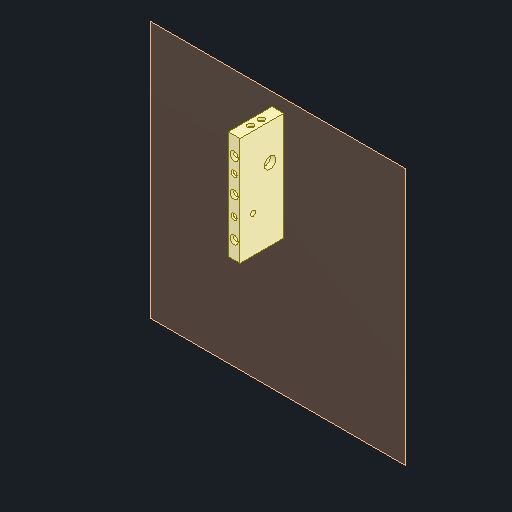
# Autodesk Inventor part: middle_gear_holder
Saved by Autodesk Inventor 2023 (Build 270158000, 158)
## iProperties
Created: 2024-04-23
Part Number: middle_gear_holder
Material: Nylon 6/6
Document SubType Name: Modeling
Designer: szymo
Density: 1.13 g/cm^3
Appearance: Nylon 6
Mass: 25.6721 g
Surface Area: 95.1123 cm^2
Volume: 22.7187 cm^3
Author: szymo
Autodesk Inventor part; units mm, degrees
ref_plane "YZ Plane" through (0, 0, 0) normal (1, 0, 0) x (0, 1, 0)
ref_plane "XZ Plane" through (0, 0, 0) normal (0, 1, 0) x (-1, 0, 0)
ref_plane "XY Plane" through (0, 0, 0) normal (0, 0, 1) x (1, 0, 0)
ref_plane "Work Plane1" through (0, 0, 0) normal (0, 0, 1) x (1, 0, 0)
ref_plane "Work Plane2" through (-89, -40.3889, 33.5) normal (0, 0, 1) x (1, 0, 0)
sketch "Sketch1" plane through (0, 0, 0) normal (0, 0, 1) x (1, 0, 0)
  line L0 (23.5, 88.5) -> (-23.5, 88.5) projected
  line L1 (-23.5, 88.5) -> (-23.5, 36.5) projected
  line L2 (-26.5, 33.5) -> (-89, 33.5) projected
  line L3 (-89, 33.5) -> (-89, -72.5) projected
  line L4 (-89, -72.5) -> (-77, -72.5) projected
  line L5 (-74, -75.5) -> (-74, -93.5) projected
  line L6 (-74, -93.5) -> (74, -93.5) projected
  line L7 (74, -93.5) -> (74, -75.5) projected
  line L8 (77, -72.5) -> (89, -72.5) projected
  line L9 (89, -72.5) -> (89, 33.5) projected
  line L10 (89, 33.5) -> (26.5, 33.5) projected
  line L11 (23.5, 36.5) -> (23.5, 88.5) projected
  line L12 (-4.5, 81.5) -> (-4.5, 36.5) projected
  line L13 (-7.5, 33.5) -> (-13.5, 33.5) projected
  line L14 (-16.5, 36.5) -> (-16.5, 81.5) projected
  line L15 (7.5, 84.5) -> (13.5, 84.5) projected
  line L16 (16.5, 81.5) -> (16.5, 36.5) projected
  line L17 (13.5, 33.5) -> (7.5, 33.5) projected
  line L18 (4.5, 36.5) -> (4.5, 81.5) projected
  line L19 (-13.5, 84.5) -> (-7.5, 84.5) projected
  line L20 (-4.5, 88.5) -> (4.5, 88.5)
  line L21 (4.5, 88.5) -> (4.5, 5.75)
  line L22 (4.5, 5.75) -> (-4.5, 5.75)
  line L23 (-4.5, 5.75) -> (-4.5, 88.5)
  line L24 (-32.2, 4.75) -> (-59.9, 4.75)
  arc A0 (13.5, 33.5) -> (16.5, 36.5) centre (13.5, 36.5) ccw projected
  arc A1 (4.5, 36.5) -> (7.5, 33.5) centre (7.5, 36.5) ccw projected
  arc A2 (7.5, 84.5) -> (4.5, 81.5) centre (7.5, 81.5) ccw projected
  arc A3 (16.5, 81.5) -> (13.5, 84.5) centre (13.5, 81.5) ccw projected
  arc A4 (-4.5, 81.5) -> (-7.5, 84.5) centre (-7.5, 81.5) ccw projected
  arc A5 (-7.5, 33.5) -> (-4.5, 36.5) centre (-7.5, 36.5) ccw projected
  arc A6 (-16.5, 36.5) -> (-13.5, 33.5) centre (-13.5, 36.5) ccw projected
  arc A7 (-13.5, 84.5) -> (-16.5, 81.5) centre (-13.5, 81.5) ccw projected
  arc A8 (-26.5, 33.5) -> (-23.5, 36.5) centre (-26.5, 36.5) ccw projected
  arc A9 (-74, -75.5) -> (-77, -72.5) centre (-77, -75.5) ccw projected
  arc A10 (77, -72.5) -> (74, -75.5) centre (77, -75.5) ccw projected
  arc A11 (23.5, 36.5) -> (26.5, 33.5) centre (26.5, 36.5) ccw projected
  circle A12 centre (39.125, 25.9125) radius 1.0065 projected
  circle A13 centre (72.95, 12.275) radius 1.0065 projected
  circle A14 centre (86, 30.5) radius 1.0065 projected
  circle A15 centre (-86, 30.5) radius 1.0065 projected
  circle A16 centre (-39.125, 12.3375) radius 1.0065 projected
  circle A17 centre (-72.95, 25.975) radius 1.0065 projected
  circle A18 centre (-72.95, 12.275) radius 1.0065 projected
  circle A19 centre (-39.125, 25.9125) radius 1.0065 projected
  circle A20 centre (-86, 7.75) radius 1.0065 projected
  circle A21 centre (86, 7.75) radius 1.0065 projected
  circle A22 centre (72.95, 25.975) radius 1.0065 projected
  circle A23 centre (39.125, 12.3375) radius 1.0065 projected
  circle A24 centre (-24.1, -73.1) radius 1.2295 projected
  circle A25 centre (-42.4984, -44.6666) radius 1.2295 projected
  circle A26 centre (-79, -42.3889) radius 1.2295 projected
  circle A27 centre (-19.5, 28.875) radius 1.2295 projected
  circle A28 centre (19.5, 9.55) radius 1.2295 projected
  circle A29 centre (19.5, 47.3) radius 1.2295 projected
  circle A30 centre (-19.5, 47.3) radius 1.2295 projected
  circle A31 centre (0, 74.7) radius 1.2295 projected
  circle A32 centre (-19.4231, 74.8077) radius 1.2295 projected
  circle A33 centre (19.5, 74.7) radius 1.2295 projected
  circle A34 centre (0, 49.05) radius 1.2295 projected
  circle A35 centre (19.5, 28.875) radius 1.2295 projected
  circle A36 centre (0, 19.125) radius 1.2295 projected
  circle A37 centre (-19.5, 9.55) radius 1.2295 projected
  circle A38 centre (24.1, -73.1) radius 1.2295 projected
  circle A39 centre (42.5, -44.6649) radius 1.2295 projected
  circle A40 centre (79, -42.3889) radius 1.2295 projected
  circle A41 centre (21.5, -85.5) radius 1.8 projected
  circle A42 centre (-64.5, -85.5) radius 1.8 projected
  circle A43 centre (-83.4, -19.2889) radius 1.8 projected
  circle A44 centre (-21.5, -85.5) radius 1.8 projected
  circle A45 centre (64.5, -85.5) radius 1.8 projected
  line L25 (-58.2315, -77.6013) -> (-77.7685, -63.3434) projected
  line L26 (-79, -36.3889) -> (-79, 1.75) projected
  line L27 (-75.7766, -45.4056) -> (-47.1423, -47.5438) projected
  line L28 (-21.1, -26.5751) -> (-21.1, -22.0255) projected
  line L29 (-46.9357, -41.5592) -> (-76, -39.3889) projected
  line L30 (-79, -60.9201) -> (-79, -48.3972) projected
  line L31 (32.0924, 4.75) -> (76, 4.75) projected
  line L32 (79, 1.75) -> (79, -36.3889) projected
  line L33 (76, -39.3889) -> (46.9371, -41.5577) projected
  line L34 (21.1, -22.0255) -> (21.1, -26.5749) projected
  line L35 (47.144, -47.5423) -> (76, -45.3889) projected
  line L36 (79, -48.3889) -> (79, -60.9201) projected
  line L37 (77.7685, -63.3434) -> (58.2315, -77.6013) projected
  line L38 (57, -80.0246) -> (57, -87.5) projected
  arc A46 (55, -89.5) -> (57, -87.5) centre (55, -87.5) ccw projected
  line L39 (55, -89.5) -> (31, -89.5) projected
  arc A47 (29, -87.5) -> (31, -89.5) centre (31, -87.5) ccw projected
  line L40 (29, -87.5) -> (29, -79.2522) projected
  line L41 (14, -79.5039) -> (14, -87.5) projected
  arc A48 (12, -89.5) -> (14, -87.5) centre (12, -87.5) ccw projected
  line L42 (12, -89.5) -> (-12, -89.5) projected
  arc A49 (-14, -87.5) -> (-12, -89.5) centre (-12, -87.5) ccw projected
  line L43 (-14, -87.5) -> (-14, -79.5039) projected
  line L44 (-29, -79.2522) -> (-29, -87.5) projected
  arc A50 (-31, -89.5) -> (-29, -87.5) centre (-31, -87.5) ccw projected
  line L45 (-31, -89.5) -> (-55, -89.5) projected
  arc A51 (-57, -87.5) -> (-55, -89.5) centre (-55, -87.5) ccw projected
  line L46 (-57, -87.5) -> (-57, -80.0246) projected
  line L47 (-66.95, 28.9125) -> (-45.125, 28.9125) projected
  line L48 (-42.125, 25.9125) -> (-42.125, 12.275) projected
  line L49 (-45.125, 9.275) -> (-66.95, 9.275) projected
  line L50 (-69.95, 12.275) -> (-69.95, 25.9125) projected
  line L51 (-16.5, 12.75) -> (-16.5, 25.5) projected
  line L52 (-13.5, 28.5) -> (-7.5, 28.5) projected
  line L53 (-4.5, 25.5) -> (-4.5, 12.75) projected
  line L54 (-7.5, 9.75) -> (-13.5, 9.75) projected
  line L55 (66.95, 9.3375) -> (45.125, 9.3375) projected
  line L56 (42.125, 12.3375) -> (42.125, 25.975) projected
  line L57 (45.125, 28.975) -> (66.95, 28.975) projected
  line L58 (69.95, 25.975) -> (69.95, 12.3375) projected
  line L59 (4.5, 12.75) -> (4.5, 25.5) projected
  line L60 (7.5, 28.5) -> (13.5, 28.5) projected
  line L61 (16.5, 25.5) -> (16.5, 12.75) projected
  line L62 (13.5, 9.75) -> (7.5, 9.75) projected
  line L63 (44.5181, -40.6102) -> (28.0046, -22.8717) projected
  line L64 (27.2109, -20.577) -> (29.1029, 2.0005) projected
  line L65 (-44.7206, -49.1201) -> (-29.3549, -77.8368) projected
  line L66 (-76, 4.75) -> (-32.0924, 4.75) projected
  line L67 (-29.1029, 2.0005) -> (-27.2109, -20.5772) projected
  line L68 (-28.0044, -22.8717) -> (-44.5164, -40.6115) projected
  line L69 (29.3549, -77.8368) -> (44.7222, -49.1185) projected
  line L70 (-14.6042, -77.6983) -> (-37.8537, -46.8489) projected
  line L71 (-37.4786, -42.8259) -> (-22.0793, -28.7924) projected
  line L72 (-21.1105, -21.775) -> (-23.0609, 1.4995) projected
  line L73 (-20.0714, 4.75) -> (20.0714, 4.75) projected
  line L74 (23.0609, 1.4995) -> (21.1105, -21.775) projected
  line L75 (22.0795, -28.7925) -> (37.4798, -42.8243) projected
  line L76 (37.8551, -46.8475) -> (14.6042, -77.6983) projected
  circle A52 centre (-78, -67.1725) radius 1.2295 projected
  arc A53 (76, -39.3889) -> (79, -36.3889) centre (76, -36.3889) ccw projected
  arc A54 (44.5181, -40.6102) -> (46.9371, -41.5577) centre (46.7138, -38.566) ccw projected
  arc A55 (27.2109, -20.577) -> (28.0046, -22.8717) centre (30.2004, -20.8276) ccw projected
  arc A56 (32.0924, 4.75) -> (29.1029, 2.0005) centre (32.0924, 1.75) ccw projected
  arc A57 (79, 1.75) -> (76, 4.75) centre (76, 1.75) ccw projected
  arc A58 (-42.125, 25.9125) -> (-45.125, 28.9125) centre (-45.125, 25.9125) ccw projected
  arc A59 (-45.125, 9.275) -> (-42.125, 12.275) centre (-45.125, 12.275) ccw projected
  arc A60 (-69.95, 12.275) -> (-66.95, 9.275) centre (-66.95, 12.275) ccw projected
  arc A61 (-66.95, 28.9125) -> (-69.95, 25.9125) centre (-66.95, 25.9125) ccw projected
  arc A62 (-13.5, 28.5) -> (-16.5, 25.5) centre (-13.5, 25.5) ccw projected
  arc A63 (-4.5, 25.5) -> (-7.5, 28.5) centre (-7.5, 25.5) ccw projected
  arc A64 (-7.5, 9.75) -> (-4.5, 12.75) centre (-7.5, 12.75) ccw projected
  arc A65 (-16.5, 12.75) -> (-13.5, 9.75) centre (-13.5, 12.75) ccw projected
  arc A66 (58.2315, -77.6013) -> (57, -80.0246) centre (60, -80.0246) ccw projected
  arc A67 (29.3549, -77.8368) -> (29, -79.2522) centre (32, -79.2522) ccw projected
  arc A68 (47.144, -47.5423) -> (44.7222, -49.1185) centre (47.3673, -50.5339) ccw projected
  arc A69 (79, -48.3889) -> (76, -45.3889) centre (76, -48.3889) ccw projected
  arc A70 (77.7685, -63.3434) -> (79, -60.9201) centre (76, -60.9201) ccw projected
  arc A71 (-21.1, -22.0255) -> (-21.1105, -21.775) centre (-24.1, -22.0255) ccw projected
  arc A72 (-20.0714, 4.75) -> (-23.0609, 1.4995) centre (-20.0714, 1.75) ccw projected
  arc A73 (23.0609, 1.4995) -> (20.0714, 4.75) centre (20.0714, 1.75) ccw projected
  arc A74 (21.1105, -21.775) -> (21.1, -22.0255) centre (24.1, -22.0255) ccw projected
  arc A75 (21.1, -26.5749) -> (22.0795, -28.7925) centre (24.1, -26.5749) ccw projected
  arc A76 (37.8551, -46.8475) -> (37.4798, -42.8243) centre (35.4593, -45.0419) ccw projected
  arc A77 (14.6042, -77.6983) -> (14, -79.5039) centre (17, -79.5039) ccw projected
  arc A78 (-14, -79.5039) -> (-14.6042, -77.6983) centre (-17, -79.5039) ccw projected
  arc A79 (-37.4786, -42.8259) -> (-37.8537, -46.8489) centre (-35.4579, -45.0433) ccw projected
  arc A80 (-22.0793, -28.7924) -> (-21.1, -26.5751) centre (-24.1, -26.5751) ccw projected
  arc A81 (-79, -36.3889) -> (-76, -39.3889) centre (-76, -36.3889) ccw projected
  arc A82 (-76, 4.75) -> (-79, 1.75) centre (-76, 1.75) ccw projected
  arc A83 (-29.1029, 2.0005) -> (-32.0924, 4.75) centre (-32.0924, 1.75) ccw projected
  arc A84 (-28.0044, -22.8717) -> (-27.2109, -20.5772) centre (-30.2004, -20.8277) ccw projected
  arc A85 (-46.9357, -41.5592) -> (-44.5164, -40.6115) centre (-46.7123, -38.5676) ccw projected
  arc A86 (7.5, 28.5) -> (4.5, 25.5) centre (7.5, 25.5) ccw projected
  arc A87 (16.5, 25.5) -> (13.5, 28.5) centre (13.5, 25.5) ccw projected
  arc A88 (13.5, 9.75) -> (16.5, 12.75) centre (13.5, 12.75) ccw projected
  arc A89 (4.5, 12.75) -> (7.5, 9.75) centre (7.5, 12.75) ccw projected
  arc A90 (-57, -80.0246) -> (-58.2315, -77.6013) centre (-60, -80.0246) ccw projected
  arc A91 (-79, -60.9201) -> (-77.7685, -63.3434) centre (-76, -60.9201) ccw projected
  arc A92 (-75.7766, -45.4056) -> (-79, -48.3972) centre (-76, -48.3972) ccw projected
  arc A93 (-44.7206, -49.1201) -> (-47.1423, -47.5438) centre (-47.3657, -50.5355) ccw projected
  arc A94 (-29, -79.2522) -> (-29.3549, -77.8368) centre (-32, -79.2522) ccw projected
  arc A95 (42.125, 12.3375) -> (45.125, 9.3375) centre (45.125, 12.3375) ccw projected
  arc A96 (45.125, 28.975) -> (42.125, 25.975) centre (45.125, 25.975) ccw projected
  arc A97 (69.95, 25.975) -> (66.95, 28.975) centre (66.95, 25.975) ccw projected
  arc A98 (66.95, 9.3375) -> (69.95, 12.3375) centre (66.95, 12.3375) ccw projected
  circle A99 centre (83.4, -16.3889) radius 1.8 projected
  circle A100 centre (78, -67.1725) radius 1.2295 projected
  circle A101 centre (24.1, -24.9) radius 1.2295 projected
  circle A102 centre (-24.1, -24.9) radius 1.2295 projected
  point P0 (0, 0)
  point P1 (-4.5, 81.5)
  point P2 (-4.5, 36.5)
  point P3 (7.5, 81.5)
  point P4 (13.5, 81.5)
  point P5 (-7.5, 81.5)
  point P6 (-13.5, 81.5)
  point P7 (39, -44.2094)
  point P8 (-4.5, 28.5)
  point P9 (-4.5, 9.75)
  point P10 (4.5, 9.75)
  point P11 (4.5, 28.5)
  point P12 (-79, -67.8878)
  point P13 (-79, -66.4572)
  dimension "d41" = 1
  constraints: 10 end point, 2 collinear, 2 horizontal, 2 parallel, 1 perpendicular, 1 point on line, 2 other
  measures "d41" distance between parallel lines of L22 L24
extrude "Extrusion1" add sketch "Sketch1" along normal up to surface (33.5 mm away) contours L21 L18 L22 L23 L12 L0 | A31 | A34 | A36
sketch "Sketch2" plane through (4.5, 5.75, 0) normal (1, 0, 0) x (0, 0, -1)
  circle A0 centre (-23.4363, 28.1825) radius 2 projected
  point P0 (0, -5.75)
extrude "Extrusion2" cut sketch "Sketch2" against normal blind 10
sketch "Sketch3" plane through (4.5, 5.75, 0) normal (1, 0, 0) x (0, 0, -1)
  circle A0 centre (-10.5, 55.25) radius 4.5 projected
  point P0 (0, -5.75)
extrude "Extrusion3" cut sketch "Sketch3" against normal blind 4
sketch "Sketch4" plane through (-4.5, 5.75, 0) normal (-1, 0, 0) x (0, 0, 1)
  circle A0 centre (10.5, 55.25) radius 4.5 projected
  point P0 (0, -5.75)
extrude "Extrusion4" cut sketch "Sketch4" against normal blind 4
sketch "Sketch5" plane through (-4.5, 5.75, 33.5) normal (0, 0, 1) x (1, 0, 0)
  line L0 (5, 59.75) -> (5, 50.75) projected
  line L1 (4, 50.75) -> (4, 59.75) projected
  line L2 (9, 26.1825) -> (0, 26.1825) projected
  line L3 (9, 30.1825) -> (0, 30.1825) projected
  line L4 (17, 78.15) -> (-8, 78.15)
  line L5 (-8, 35.85) -> (17, 35.85)
  line L6 (9, 82.75) -> (9, 0) projected
  line L7 (0, 50.75) -> (0, 59.75) projected
  line L8 (9, 35.85) -> (0, 35.85)
  line L9 (0, 35.85) -> (0, 50.75)
  line L10 (0, 50.75) -> (9, 50.75)
  line L11 (9, 50.75) -> (9, 35.85)
  line L12 (0, 0) -> (0, 82.75) projected
  line L13 (9, 78.15) -> (0, 78.15)
  line L14 (0, 78.15) -> (0, 59.75)
  line L15 (0, 59.75) -> (9, 59.75)
  line L16 (9, 59.75) -> (9, 78.15)
  line L17 (-18, 6.625) -> (-18, 20.125) projected
  line L18 (-18, 13.375) -> (27, 13.375)
  line L19 (9, 35.85) -> (0, 50.75)
  line L20 (9, 59.75) -> (9, 50.75) projected
  line L21 (0, 35.85) -> (9, 50.75)
  line L22 (9, 59.75) -> (0, 78.15)
  line L23 (0, 59.75) -> (9, 78.15)
  point P0 (4.5, -5.75)
  point P1 (4.5, 13.375)
  point P2 (4.5, 43.3)
  point P3 (4.5, 68.95)
  dimension "d9" = 4.5
  dimension "d10" = 4.5
  constraints: 30 end point, 5 horizontal, 5 point on line, 4 midpoint, 4 parallel, 2 perpendicular, 4 other
  measures "d9" distance from line of L6 point (4.5, 13.375)
  measures "d10" distance from line of point (4.5, 13.375) L12
hole "Hole1" at (0, 19.125, 33.5) at (0, 49.05, 33.5) at (0, 74.7, 33.5) direction (0, 0, -1) diameter 3.6 end through all countersink diameter 6.6 countersink angle 90 clearance for "Countersunk Flat Head Screw ISO 2009/7046" size "M3" standard "ISO"
sketch "Sketch6" plane through (-4.5, 5.75, 0) normal (0, -1, 0) x (1, 0, 0)
  line L0 (9, 33.5) -> (0, 33.5) projected
  line L1 (0, 0) -> (0, 33.5) projected
  line L2 (0, 0) -> (9, 0) projected
  line L3 (9, 0) -> (9, 33.5) projected
  line L4 (0, 16.75) -> (9, 16.75)
  line L5 (9, 16.75) -> (0, 33.5)
  line L6 (9, 33.5) -> (0, 16.75)
  line L7 (0, 16.75) -> (9, 0)
  line L8 (9, 16.75) -> (0, 0)
  point P0 (4.5, 0)
  point P1 (4.5, 8.375)
  point P2 (4.5, 25.125)
  constraints: 10 end point, 4 midpoint, 2 parallel
hole "Hole2" at (0, 5.75, 8.375) at (0, 5.75, 25.125) direction (0, 1, 0) diameter 4 depth 6.6 counterbore diameter 5 counterbore depth 2
sketch "Sketch7" plane through (-4.5, 88.5, 0) normal (0, 1, 0) x (1, 0, 0)
  line L0 (0, -33.5) -> (9, -33.5) projected
  line L1 (0, -33.5) -> (9, -33.5) projected
  line L2 (9, 0) -> (9, -33.5) projected
  line L3 (9, 0) -> (0, 0) projected
  line L4 (0, 0) -> (0, -33.5) projected
  line L5 (-8, -1.4) -> (-8, -6.6) projected
  line L6 (-8, -32.1) -> (-8, -26.9) projected
  line L7 (17, -32.1) -> (17, -26.9) projected
  line L8 (17, -1.4) -> (17, -6.6) projected
  line L9 (17, -32.1) -> (-8, -32.1)
  line L10 (-8, -32.1) -> (-8, -26.9)
  line L11 (-8, -26.9) -> (17, -26.9)
  line L12 (17, -26.9) -> (17, -32.1)
  line L13 (-8, -6.6) -> (17, -6.6)
  line L14 (17, -6.6) -> (17, -1.4)
  line L15 (17, -1.4) -> (-8, -1.4)
  line L16 (-8, -1.4) -> (-8, -6.6)
  line L17 (17, -6.6) -> (-8, -6.6)
  line L18 (-8, -6.6) -> (-8, -8.6)
  line L19 (-8, -8.6) -> (17, -8.6)
  line L20 (17, -8.6) -> (17, -6.6)
  line L21 (-8, -26.9) -> (17, -26.9)
  line L22 (17, -26.9) -> (17, -24.9)
  line L23 (17, -24.9) -> (-8, -24.9)
  line L24 (-8, -24.9) -> (-8, -26.9)
  line L25 (9, 0) -> (9, -33.5) projected
  line L26 (9, -16.75) -> (0, -16.75)
  line L27 (0, 0) -> (0, -33.5) projected
  line L28 (9, -24.9) -> (0, -16.75)
  line L29 (9, -8.6) -> (0, -16.75)
  line L30 (0, -8.6) -> (9, -16.75)
  line L31 (9, -16.75) -> (0, -24.9)
  point P0 (4.5, 0)
  point P1 (4.5, -20.825)
  point P2 (4.5, -12.675)
  dimension "d25" = 2
  dimension "d26" = 2
  constraints: 42 end point, 10 point on line, 8 parallel, 5 midpoint, 4 horizontal, 4 perpendicular
  measures "d25" distance of L18.end L17.end
  measures "d26" distance of L22.end L21.end
hole "Hole3" at (0, 88.5, 20.825) at (0, 88.5, 12.675) direction (0, -1, 0) diameter 4 depth 6.5 counterbore diameter 4.6 counterbore depth 2
sketch "Sketch8" plane through (-4.5, 5.75, 33.5) normal (0, 0, 1) x (1, 0, 0)
  line L0 (26, 27.2497) -> (-17, 27.2497)
  line L1 (26, 31.2497) -> (-17, 31.2497)
  line L2 (4, 52.75) -> (-1, 52.75)
  line L3 (4, 61.75) -> (-1, 61.75)
  line L4 (10, 61.75) -> (5, 61.75)
  line L5 (9, 50.75) -> (5, 50.75) projected
  line L6 (0, 0) -> (0, 82.75) projected
  line L7 (9, 52.75) -> (0, 52.75)
  line L8 (0, 52.75) -> (0, 61.75)
  line L9 (0, 61.75) -> (9, 61.75)
  line L10 (9, 61.75) -> (9, 50.75)
  line L11 (9, 26.1825) -> (0, 26.1825) projected
  line L12 (0, 31.2497) -> (9, 31.2497)
  line L13 (9, 31.2497) -> (9, 26.1825)
  line L14 (9, 26.1825) -> (0, 26.1825)
  line L15 (0, 26.1825) -> (0, 31.2497)
  line L16 (9, 26.1825) -> (0, 31.2497)
  line L17 (0, 26.1825) -> (9, 31.2497)
  line L18 (10, 51.75) -> (0, 61.75)
  line L19 (0, 52.75) -> (9, 61.75)
  point P0 (4.5, -5.75)
  point P1 (4.5, 28.7161)
  point P2 (4.5, 57.25)
  constraints: 34 end point, 7 horizontal, 6 point on line, 4 parallel, 3 perpendicular, 2 midpoint, 10 other
hole "Hole4" at (0, 34.4661, 33.5) at (0, 63, 33.5) direction (0, 0, -1) diameter 4 depth 6 counterbore diameter 4.6 counterbore depth 1.5
equation "\"d9\" = d10"
body "Solid1"
